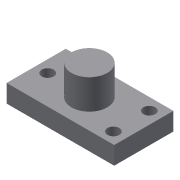
# Autodesk Inventor part: Основание БЕЗ опор по бокам
Saved by Autodesk Inventor 2014 SP1 (Build 180222100, 222)
## iProperties
Created: 2023-10-15
Part Number: Основание БЕЗ опор по бокам
Material: Типовые
Document SubType Name: Modeling
Designer: Konstantin
Density: 1 g/cm^3
Appearance: По умолчанию
Author: Konstantin
Autodesk Inventor part; units mm, degrees
ref_plane "YZ Plane" through (0, 0, 0) normal (1, 0, 0) x (0, 1, 0)
ref_plane "XZ Plane" through (0, 0, 0) normal (0, 1, 0) x (-1, 0, 0)
ref_plane "XY Plane" through (0, 0, 0) normal (0, 0, 1) x (1, 0, 0)
sketch "Эскиз4" plane through (0, 0, 0) normal (0, 0, 1) x (1, 0, 0)
  line L0 (45.2395, 25.2453) -> (-44.981, 25.2453)
  line L1 (-44.981, 25.2453) -> (-44.981, -24.4084)
  line L2 (-44.981, -24.4084) -> (45.2395, -24.4084)
  line L3 (45.2395, -24.4084) -> (45.2395, 25.2453)
  point P0 (0, 0)
  constraints: 8 end point, 2 parallel, 1 horizontal, 1 perpendicular
extrude "Прямоугольник_" add sketch "Эскиз4" along normal blind 15
sketch "Прямоугольник" plane through (0, 0, 0) normal (0, 0, 1) x (1, 0, 0)
  line L0 (-77.4921, 158.0418) -> (133.4103, 158.0418) construction
  line L1 (133.4103, 158.0418) -> (133.4103, -71.9132) construction
  line L2 (133.4103, -71.9132) -> (-77.4921, -71.9132) construction
  line L3 (-77.4921, -71.9132) -> (-77.4921, 158.0418) construction
  line L4 (44.9907, 25.2614) -> (-45.0093, 25.2614)
  line L5 (-45.0093, 25.2614) -> (-45.0093, -24.7386)
  line L6 (-45.0093, -24.7386) -> (44.9907, -24.7386)
  line L7 (44.9907, -24.7386) -> (44.9907, 25.2614)
  point P0 (0, 0)
  dimension "d17" = 90
  dimension "d20" = 50
  constraints: 8 end point, 2 parallel, 1 horizontal, 1 perpendicular, 2 other
  measures "d17" distance of L4.start L4.end
  measures "d20" distance of L6.end L4.start
sketch "Три отверстия по краям" plane through (0, 0, 15) normal (0, 0, 1) x (1, 0, 0)
  circle A0 centre (-34.9124, 0) radius 5
  circle A1 centre (35.035, 15.2594) radius 5
  circle A2 centre (35.035, -14.8643) radius 5
  point P0 (0, 0)
  dimension "d12" = 10
  dimension "d13" = 10
  dimension "d14" = 10
  constraints: 3 centre point
  measures "d12" diameter of A0
  measures "d13" diameter of A1
  measures "d14" diameter of A2
extrude "3 отверстия по краям" cut sketch "Три отверстия по краям" against normal blind 800
sketch "Возвышенность по центру" plane through (0, 0, 15) normal (0, 0, 1) x (1, 0, 0)
  circle A0 centre (0, 0) radius 15
  dimension "d21" = 30
  constraints: 1 centre point, 1 coincident
  measures "d21" diameter of A0
extrude "Возвышенность" add sketch "Возвышенность по центру" along normal blind 25
sketch "Эскиз7" plane through (0, 0, 0) normal (0, 0, -1) x (-1, 0, 0)
  circle A0 centre (0, 0) radius 9
  dimension "d24" = 18
  constraints: 1 centre point, 1 coincident
  measures "d24" diameter of A0
extrude "Внутренняя часть внутри возв" cut sketch "Эскиз7" against normal blind 38
